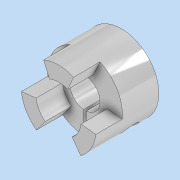
# Autodesk Inventor part: PHAN NHOM
Saved by Autodesk Inventor 2021 (Build 250183000, 183)
## iProperties
Created: 2022-03-09
Part Number: PHAN NHOM
Material: Generic
Document SubType Name: Modeling
Designer: 41601100
Density: 1 g/cm^3
Appearance: Default
Author: 41601100
Autodesk Inventor part; units mm, degrees
ref_plane "XZ Plane" through (0, 0, 0) normal (0, 1, 0) x (-1, 0, 0)
ref_plane "XY Plane" through (0, 0, 0) normal (0, 0, 1) x (1, 0, 0)
sketch "Sketch1" plane through (0, 0, 0) normal (0, 0, 1) x (1, 0, 0)
  circle A0 centre (0, 0) radius 14.89
  circle A1 centre (0, 0) radius 6
  circle A2 centre (0, 0) radius 3.175
  dimension "d0" = 29.78
  dimension "d1" = 12
  dimension "d41" = 6.35
  constraints: 3 centre point, 3 coincident
  measures "d0" diameter of A0
  measures "d1" diameter of A1
  measures "d41" diameter of A2
extrude "Extrusion1" add sketch "Sketch1" along normal blind 25 contours A0
sketch "Sketch2" plane through (0, 0, 25) normal (0, 0, 1) x (1, 0, 0)
  circle A0 centre (0, 0) radius 14.89 projected
  circle A1 centre (0, 0) radius 9
  circle A2 centre (0, 0) radius 14.89 projected
  line L0 (-3.6007, 8.2483) -> (-5.9571, 13.6464)
  line L1 (5.9571, 13.6464) -> (3.6007, 8.2483)
  line L2 (-5.3429, -7.2425) -> (-8.8396, -11.9822)
  line L3 (-14.7967, -1.6642) -> (-8.9436, -1.0059)
  line L4 (8.9436, -1.0059) -> (14.7967, -1.6642)
  line L5 (8.8396, -11.9822) -> (5.3429, -7.2425)
  dimension "d14" = 18
  dimension "d24" = 360
  constraints: 12 end point, 4 point on circle, 1 centre point, 19 other
  measures "d14" diameter of A1
extrude "Extrusion2" cut sketch "Sketch2" against normal blind 10.5 contours A0 L4 A1 L1 | L0 A1 L3 A0 | A1 | A0 L2 A1 L5
ref_plane "Work Plane1" through (14.9, 0, 0) normal (1, 0, 0) x (0, 1, 0)
sketch "Sketch3" plane through (14.9, 0, 0) normal (1, 0, 0) x (0, 1, 0)
  line L0 (-1.6642, 14.5) -> (-1.6642, 25) projected
  line L1 (-11.9822, 25) -> (-1.6642, 25) projected
  line L2 (-11.9822, 25) -> (-11.9822, 14.5) projected
  line L3 (-11.9822, 14.5) -> (-11.9822, 14.5) projected
  line L4 (-11.9822, 14.5) -> (-11.9822, 25) projected
  line L5 (-1.6642, 25) -> (-11.9822, 25) projected
  line L6 (-1.6642, 25) -> (-1.6642, 14.5) projected
  line L7 (-1.6642, 14.5) -> (13.6464, 14.5) projected
  line L8 (13.6464, 14.5) -> (13.6464, 25) projected
  line L9 (13.6464, 25) -> (13.6464, 25) projected
  line L10 (13.6464, 25) -> (13.6464, 14.5) projected
  line L11 (13.6464, 14.5) -> (-1.6642, 14.5) projected
  line L12 (14.89, 0) -> (-14.89, 0) projected
  line L13 (14.89, 25) -> (13.6464, 25) projected
  line L14 (14.89, 25) -> (14.89, 0)
  line L15 (14.89, 0) -> (14.89, 25) projected
  line L16 (-14.89, 0) -> (-14.89, 14.5) projected
  line L17 (14.89, 0) -> (-14.89, 0) projected
  line L18 (-14.89, 14.5) -> (-14.89, 0)
  line L19 (-7.89, 0) -> (-14.89, 0)
  line L20 (-14.89, 0) -> (-14.89, 14.5)
  line L21 (-14.89, 7.25) -> (-7.89, 7.25)
  circle A0 centre (-11.39, 7.25) radius 3.5
  circle A1 centre (-11.39, 7.25) radius 1.75
  point P0 (0, 0)
  dimension "d27" = 29.78
  dimension "d30" = 3.5
  constraints: 10 end point, 2 midpoint, 2 perpendicular, 1 centre point, 1 coincident, 1 collinear, 1 horizontal alignment, 1 point on line, 1 vertical, 2 other
  measures "d27" distance of L15.start L19.end
  measures "d30" diameter of A1
extrude "Extrusion3" cut sketch "Sketch3" against normal blind 10
extrude "Extrusion4" cut sketch "Sketch3" against normal blind 30 contours A1 L21 | L21 A1
sketch "Sketch4" plane through (0, 0, 0) normal (0, 0, -1) x (-1, 0, 0)
  arc A0 (-8.8396, -11.9822) -> (8.8396, -11.9822) centre (0, 0) ccw projected
  line L0 (0, 0) -> (-0.5, 0)
  line L1 (-0.5, 0) -> (-0.5, -14.8816)
  line L2 (0, 0) -> (0.5, 0)
  line L3 (0.5, 0) -> (0.5, -14.8816)
  line L4 (-0.5, 0) -> (-0.5, 14.8816)
  line L5 (0.5, 0) -> (0.5, 14.8816)
  arc A1 (5.3429, -7.2425) -> (8.9436, -1.0059) centre (0, 0) ccw projected
  circle A2 centre (0, 0) radius 14.89 projected
  point P0 (-8.8396, 11.9822)
  dimension "d33" = 0.5
  dimension "d34" = 0.5
  constraints: 12 end point, 3 symmetric about line, 2 horizontal, 2 perpendicular, 2 point on circle
  measures "d33" distance of L0.start L0.end
  measures "d34" distance of L0.start L2.end
extrude "Extrusion5" cut sketch "Sketch4" against normal blind 15 contours L1 L0 L2 L3 A0
sketch "Sketch5" plane through (-0.5, -14.8816, 0) normal (1, 0, 0) x (0, 0, -1)
  line L0 (0, 0) -> (-14.5, 0) projected
  line L1 (-14.5, 0) -> (-14.5, 2.8994) projected
  line L2 (-14.5, 2.8994) -> (-25, 2.8994) projected
  line L3 (-25, 13.2174) -> (-25, 2.8994) projected
  line L4 (-25, 13.2174) -> (-14.5, 13.2174) projected
  line L5 (-14.5, 13.2174) -> (-14.5, 28.528) projected
  line L6 (-14.5, 28.528) -> (-25, 28.528) projected
  line L7 (-25, 28.528) -> (-25, 28.528) projected
  line L8 (-25, 28.528) -> (-14.5, 28.528) projected
  line L9 (-14.5, 28.528) -> (-14.5, 13.2174) projected
  line L10 (-14.5, 13.2174) -> (-25, 13.2174) projected
  line L11 (-25, 2.8994) -> (-25, 13.2174) projected
  line L12 (-25, 2.8994) -> (-14.5, 2.8994) projected
  line L13 (-14.5, 2.8994) -> (-14.5, 0) projected
  line L14 (-14.5, 0) -> (0, 0) projected
  line L15 (0, 0) -> (0, 0) projected
  line L16 (-4.9878, 0.8209) -> (-9.5122, 0.8209) projected
  line L17 (-14.5, 8.9025) -> (0, 8.9025) projected
  line L18 (0, 8.9025) -> (0, 8.9025) projected
  line L19 (0, 8.9025) -> (-14.5, 8.9025) projected
  line L20 (-14.5, 8.9025) -> (-14.5, 8.9025) projected
  line L21 (-14.5, 20.8816) -> (-14.5, 8.9025) projected
  line L22 (-14.5, 20.8816) -> (0, 20.8816)
  line L23 (0, 29.7716) -> (0, 0) projected
  line L24 (-14.5, 20.8816) -> (-14, 20.8816)
  line L25 (0, 29.7716) -> (0, 29.2716)
  line L26 (0, 29.2716) -> (-14, 20.8816)
  line L27 (-14.5, 20.8585) -> (0, 20.8585)
  line L28 (0, 8.9025) -> (0, 20.8816) projected
  line L29 (-14, 20.8816) -> (-14.0385, 20.8585)
  line L30 (-14.5, 18.0566) -> (0, 18.0566) projected
  line L31 (-14.5, 18.0566) -> (-14.5, 11.7462) projected
  line L32 (-14.5, 18.0145) -> (0, 18.0145)
  line L33 (-14.5, 18.0145) -> (-14, 18.0145)
  line L34 (-14, 18.0145) -> (0, 29.2716)
  point P0 (0, 14.8816)
  point P1 (-7.25, 1.7416)
  point P2 (-13.9476, 18.0566)
  dimension "d37" = 0.5
  dimension "d38" = 0.5
  dimension "d42" = 0.5
  constraints: 18 end point, 7 point on line, 3 horizontal, 1 horizontal alignment, 4 other
  measures "d37" distance of L21.start L24.end
  measures "d38" distance of L25.start L25.end
  measures "d42" distance of L32.start L33.end
extrude "Extrusion6" cut sketch "Sketch5" along normal blind 1 contours L32 L34 L30 L23 | L30 L34 L27 L23 | L32 L5 L30 L34 | L27 L34 L22 L23 | L30 L5 L27 L34 | L22 L34 L23 | L27 L29 L22 L34 | L22 L26 L34
body "Solid1"
